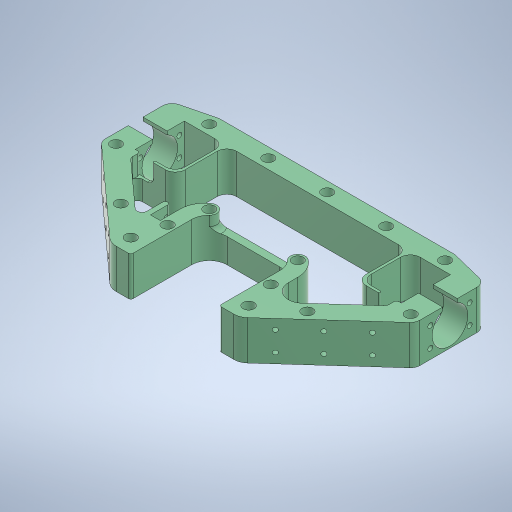
# Autodesk Inventor part: Chassis
Saved by Autodesk Inventor 2023.2 (Build 272271000, 271)
## iProperties
Created: 2022-05-26
Part Number: Chassis
Material: Nylon 6/6
Document SubType Name: Modeling
Designer: Nathan Cai
Density: 0.861189 g/cm^3
Appearance: Smooth - Dark Sea Green
Mass: 131.31 g
Surface Area: 564.609 cm^2
Volume: 152.475 cm^3
Author: Nathan Cai
Autodesk Inventor part; units mm, degrees
ref_plane "YZ Plane" through (0, 0, 0) normal (1, 0, 0) x (0, 1, 0)
ref_plane "XZ Plane" through (0, 0, 0) normal (0, 1, 0) x (-1, 0, 0)
ref_plane "XY Plane" through (0, 0, 0) normal (0, 0, 1) x (1, 0, 0)
sketch "Sketch1" plane through (0, 0, 0) normal (0, 1, 0) x (-1, 0, 0)
  line L0 (101.6, 38.1) -> (-101.6, 38.1) construction
  line L1 (-101.6, 38.1) -> (-101.6, -38.1) construction
  line L2 (-101.6, -38.1) -> (101.6, -38.1)
  line L3 (101.6, -38.1) -> (101.6, 38.1) construction
  line L4 (101.6, 38.1) -> (-101.6, -38.1) construction
  line L5 (-101.6, 38.1) -> (101.6, -38.1) construction
  line L6 (-28.575, 66.675) -> (28.575, 66.675) construction
  line L7 (28.575, 66.675) -> (28.575, 9.525)
  line L8 (28.575, 9.525) -> (-28.575, 9.525)
  line L9 (-28.575, 9.525) -> (-28.575, 66.675)
  line L10 (-28.575, 66.675) -> (28.575, 9.525) construction
  line L11 (28.575, 66.675) -> (-28.575, 9.525) construction
  circle A0 centre (-38.1, 50.8) radius 3.556
  line L12 (0, 38.1) -> (0, -38.1) construction
  circle A1 centre (-38.1, 50.8) radius 9.525
  line L13 (-38.1, 60.325) -> (-28.575, 60.325)
  circle A2 centre (38.1, 50.8) radius 3.556
  circle A3 centre (38.1, 50.8) radius 9.525
  line L14 (38.1, 60.325) -> (28.575, 60.325)
  circle A4 centre (-76.2, -38.1) radius 3.4925
  circle A5 centre (-95.25, 3.175) radius 3.4925
  circle A6 centre (76.2, -38.1) radius 3.4925
  circle A7 centre (95.25, 3.175) radius 3.4925
  line L15 (-101.6, -38.1) -> (-101.6, 6.35)
  line L16 (-101.6, 6.35) -> (-44.479723, 57.872818)
  line L17 (101.6, -38.1) -> (101.6, 6.35)
  line L18 (101.6, 6.35) -> (44.479723, 57.872818)
  line L19 (-42.641743, 42.427533) -> (-86.025, 3.295586)
  line L20 (-86.025, 3.295586) -> (-86.025, -38.1)
  line L21 (86.025, -38.1) -> (86.025, 3.295586)
  line L22 (86.025, 3.295586) -> (42.641743, 42.427533)
  line L23 (0, -38.1) -> (-95.25, -38.1)
  line L24 (0, -38.1) -> (95.25, -38.1) construction
  circle A8 centre (-60.325, 35.028711) radius 3.4925
  circle A9 centre (-33.3375, 31.75) radius 3.4925
  line L25 (-38.1, 0) -> (-38.1, 41.275)
  line L26 (-38.1, 0) -> (0, 0) construction
  circle A10 centre (60.325, 35.028711) radius 3.4925
  circle A11 centre (33.3375, 31.75) radius 3.4925
  line L27 (38.1, 0) -> (38.1, 41.275)
  line L28 (38.1, 0) -> (0, 0) construction
  line L29 (-86.025, 0) -> (-60.1, 0)
  line L30 (-60.1, 0) -> (-60.1, -31.75)
  line L31 (-60.1, -31.75) -> (-87.975, -31.75)
  line L32 (-101.6, -38.1) -> (101.6, -38.1) construction
  line L33 (101.6, -38.1) -> (101.6, 19.05)
  line L34 (101.6, 19.05) -> (-101.6, 19.05) construction
  line L35 (-101.6, 19.05) -> (-101.6, -38.1)
  line L36 (-101.6, 19.05) -> (-87.520267, 19.05) construction
  line L37 (87.520267, 19.05) -> (101.6, 19.05) construction
  circle A12 centre (-38.1, 0) radius 3.175 construction
  circle A13 centre (-38.1, 0) radius 6.35 construction
  circle A14 centre (38.1, 0) radius 3.175 construction
  circle A15 centre (38.1, 0) radius 6.35 construction
  circle A16 centre (28.575, 9.525) radius 3.4925
  circle A17 centre (28.575, 9.525) radius 4.7625
  arc A18 (17.077308, 9.525) -> (28.575, 21.022692) centre (17.077308, 21.022692) ccw
  circle A19 centre (-28.575, 9.525) radius 3.4925
  circle A20 centre (-28.575, 9.525) radius 4.7625
  arc A21 (-28.575, 21.022692) -> (-17.077308, 9.525) centre (-17.077308, 21.022692) ccw
  arc A22 (31.4325, 5.715) -> (38.1, 19.05) centre (21.43125, 19.05) ccw
  arc A23 (-38.1, 19.05) -> (-31.4325, 5.715) centre (-21.43125, 19.05) ccw
  line L38 (-58.5125, -38.1) -> (-58.5125, 28.112019)
  line L39 (86.025, 0) -> (60.1, 0)
  line L40 (60.1, 0) -> (60.1, -31.75)
  line L41 (60.1, -31.75) -> (87.975, -31.75)
  line L42 (58.5125, -38.1) -> (58.5125, 28.112019)
  line L43 (-28.575, 4.7625) -> (28.575, 4.7625)
  line L44 (101.6, -31.75) -> (-101.6, -31.75)
  line L45 (-101.6, -31.75) -> (-101.6, -44.45) construction
  line L46 (-101.6, -44.45) -> (101.6, -44.45)
  line L47 (101.6, -44.45) -> (101.6, -31.75) construction
  circle A24 centre (0, -38.1) radius 3.4925
  circle A25 centre (38.1, -38.1) radius 3.4925
  circle A26 centre (-38.1, -38.1) radius 3.4925
  line L48 (101.6, -38.1) -> (76.2, -44.45)
  line L49 (-101.6, -38.1) -> (-76.2, -44.45)
  line L50 (76.2, -38.1) -> (76.2, -44.45) construction
  line L51 (-76.2, -38.1) -> (-76.2, -44.45) construction
  line L52 (-58.5125, 1.5875) -> (-87.918653, 1.5875)
  line L53 (58.5125, 1.5875) -> (87.918653, 1.5875)
  line L54 (38.1, 19.05) -> (44.45, 19.05)
  line L55 (44.45, 19.05) -> (44.45, 31.75)
  line L56 (44.45, 31.75) -> (38.1, 31.75)
  line L57 (38.1, 31.75) -> (38.1, 19.05)
  line L58 (38.1, 19.05) -> (47.625, 19.05)
  line L59 (47.625, 19.05) -> (47.625, 37.932607)
  line L60 (47.625, 37.932607) -> (38.1, 37.932607) construction
  line L61 (38.1, 37.932607) -> (38.1, 19.05)
  point P0 (28.575, 38.1)
  point P1 (-28.575, 38.1)
  point P2 (28.575, 60.325)
  point P3 (44.479723, 57.872818)
  point P4 (101.6, -15.875)
  point P5 (38.1, 41.275)
  point P6 (-86.025, -31.75)
  point P7 (-101.6, 6.35)
  point P8 (101.6, 6.35)
  point P9 (31.75, 0)
  point P10 (38.1, 6.35)
  point P11 (-38.1, 6.35)
  point P12 (-31.75, 0)
  point P13 (86.025, -31.75)
  point P14 (86.025, 0)
  point P15 (58.5125, 28.112019)
  point P16 (-17.077308, 9.525)
  point P17 (-28.575, 21.022692)
  point P18 (-38.1, 19.05)
  point P19 (-31.4325, 5.715)
  point P20 (-21.850242, 0)
  point P21 (21.850242, 0)
  point P22 (-25.207404, 12.892596)
  point P23 (-28.575, 14.2875)
  point P24 (-23.8125, 9.525)
  point P25 (-28.575, 50.8)
  point P26 (25.207404, 12.892596)
  point P27 (28.575, 14.2875)
  point P28 (23.8125, 9.525)
  point P29 (28.575, 50.8)
  point P30 (25.0825, 9.525)
  point P31 (28.575, 13.0175)
  point P32 (58.5125, -31.75)
  point P33 (-58.5125, -31.75)
  point P34 (87.918653, 1.5875)
  point P35 (58.5125, 1.5875)
  point P36 (86.025, -31.75)
  point P37 (86.025, 1.5875)
  point P38 (-86.025, 1.5875)
  point P39 (-86.025, -31.75)
  point P40 (-34.6075, -38.1)
  point P41 (-41.5925, -38.1)
  point P42 (-3.4925, -38.1)
  point P43 (3.4925, -38.1)
  point P44 (41.5925, -38.1)
  point P45 (34.6075, -38.1)
  point P46 (-72.7075, -38.1)
  point P47 (-79.6925, -38.1)
  dimension "d166" = 12.7
  dimension "d169" = 22.225
  dimension "d0" = 203.2
  dimension "d1" = 76.2
  dimension "d4" = 57.15
  dimension "d6" = 7.112
  dimension "d7" = 38.1
  dimension "d8" = 19.05
  dimension "d10" = 6.985
  dimension "d11" = 6.985
  dimension "d12" = 0
  dimension "d14" = 25.4
  dimension "d15" = 6.35
  dimension "d20" = 50.8
  dimension "d21" = 41.275
  dimension "d22" = 44.45
  dimension "d24" = 12.7
  dimension "d25" = 15.575
  dimension "d26" = 12.7
  dimension "d27" = 15.575
  dimension "d31" = 6.985
  dimension "d32" = 6.985
  dimension "d33" = 6.35
  dimension "d34" = 31.75
  dimension "d35" = 4.7625
  dimension "d36" = 22.225
  dimension "d37" = 9.525
  dimension "d39" = 31.75
  dimension "d40" = 6.35
  dimension "d42" = 57.15
  dimension "d43" = 6.35
  dimension "d44" = 9.525
  dimension "d45" = 9.525
  dimension "d46" = 12.7
  dimension "d104" = 6.985
  dimension "d105" = 9.525
  dimension "d106" = 1.5875
  dimension "d123" = 88.9
  dimension "d124" = 12.7
  dimension "d125" = 6.985
  dimension "d126" = 6.985
  dimension "d127" = 38.1
  dimension "d128" = 28.575
  dimension "d134" = 1.5875
  dimension "d137" = 6.35
  dimension "d138" = 12.7
  dimension "d139" = 9.525
  dimension "d178" = 41.5
  constraints: 125 end point, 32 symmetric about line, 26 centre point, 25 point on line, 16 parallel, 16 point on circle, 11 horizontal, 9 perpendicular, 8 midpoint, 8 tangent, 7 coincident, 2 vertical, 1 collinear, 16 other
  measures "d0" distance of L2.end L1.end
  measures "d1" distance between parallel lines of L0 L2
  measures "d4" distance of L7.end L8.end
  measures "d6" diameter of A0
  measures "d7" distance from line of L12 A0.centre
  measures "d8" diameter of A1
  measures "d10" diameter of A4
  measures "d11" diameter of A5
  measures "d12" distance from line of L2 L51.start
  measures "d14" distance from line of L1 L51.start
  measures "d15" distance from line of L1 A5.centre
  measures "d20" distance between parallel lines of L8 L14
  measures "d21" vertical distance of L51.start A5.centre
  measures "d22" distance of L1.end L15.end
  measures "d24" distance between parallel lines of L16 L19
  measures "d25" distance between parallel lines of L15 L20
  measures "d26" distance between parallel lines of L18 L22
  measures "d27" distance from line of point (101.6, -15.875) L21
  measures "d31" diameter of A8
  measures "d32" diameter of A9
  measures "d33" distance from line of L16 A8.centre
  measures "d34" distance from line of L9 A8.centre
  measures "d35" distance from line of L9 A9.centre
  measures "d36" distance from line of L8 A9.centre
  measures "d37" distance between parallel lines of L9 L25
  measures "d39" distance between parallel lines of L31 L29
  measures "d40" distance between parallel lines of L23 L31
  measures "d42" distance of L33.end L32.end
  measures "d43" diameter of A12
  measures "d44" distance from line of L8 A12.centre
  measures "d45" distance from line of L9 A12.centre
  measures "d46" diameter of A13
  measures "d104" diameter of A16
  measures "d105" diameter of A17
  measures "d106" distance between parallel lines of L30 L38
  measures "d123" distance from line of L32 A1.centre
  measures "d124" distance between parallel lines of L44 L46
  measures "d125" diameter of A24
  measures "d126" diameter of A25
  measures "d127" distance of A24.centre A25.centre
  measures "d128" distance from line of L12 A16.centre
  measures "d134" distance between parallel lines of L29 L52
  measures "d137" distance of L56.end L55.end
  measures "d138" distance of L55.end L54.end
  measures "d139" distance of L60.end L59.end
  measures "d178" distance between parallel lines of L1 L30
extrude "Extrusion1" add sketch "Sketch1" along normal blind 25.4 contours L15 L44 L31 L20 L2 | L2 A4 A26 A24 A25 A6 L48 L46 L49 | L15 L16 A1 L19 L20 L31 L44 | L20 L31 L44 L38 L2 A4 | A1 | L2 L21 L41 L44 L17 | L20 L52 L38 L44 L30 L29 | L13 L9 A1 | L2 A6 L42 L44 L41 L21 | L44 L41 L21 L22 A3 L18 L17 | L38 L44 L42 L2 A25 A24 A26 | L9 A20 A23 L25 A1 | L42 L53 L21 L39 L40 L44 | A21 A20 L9 | A3 | A20 L8 A19 L9 | L9 A19 L8 A20 | A21 L8 A20 | A3 L7 L14 | L8 A17 L43 A20 | L22 L59 L58 L55 L56 L27 A3 | A3 L27 A22 A17 L7 | A18 A17 L8 | A17 L8 A16 L7 | L7 A17 A18 | A17 L7 A16 L8 | L54 L27 L56 L55
fillet "Fillet1" radius 6.35 14 edges at (60.1, 12.7, 0) (60.1, 12.7, -31.75) (101.6, 12.7, -38.1) (101.6, 12.7, 6.35) (-101.6, 12.7, 6.35) (-60.1, 12.7, -31.75) (-60.1, 12.7, 0) (-58.5125, 12.7, -31.75) (58.5125, 12.7, -31.75) (76.2, 12.7, -44.45) (-76.2, 12.7, -44.45) (-101.6, 12.7, -38.1) (58.5125, 12.7, 1.5875) (-58.5125, 12.7, 1.5875)
sketch "Sketch2" plane through (0, 25.4, 0) normal (0, 1, 0) x (1, 0, 0)
  line L0 (-38.1, -19.05) -> (-47.625, -19.05) projected
  line L1 (-38.1, -19.05) -> (-44.45, -19.05)
  line L2 (-44.45, -19.05) -> (-44.45, -31.75)
  line L3 (-44.45, -31.75) -> (-38.1, -31.75)
  line L4 (-38.1, -31.75) -> (-38.1, -19.05)
  point P0 (0, 0)
  dimension "d140" = 6.35
  dimension "d141" = 12.7
  constraints: 8 end point, 2 parallel, 1 horizontal, 1 perpendicular
  measures "d140" distance of L3.end L2.end
  measures "d141" distance of L2.end L1.end
extrude "Extrusion2" cut sketch "Sketch2" against normal blind 12.7
fillet "Fillet2" [suppressed]
sketch "Sketch3" plane through (101.6, 0, 15.875) normal (1, 0, 0) x (0, 0, -1)
  circle A0 centre (31.75, 12.7) radius 11.5
  line L0 (0, 25.4) -> (50.8, 25.4) projected
  line L1 (50.8, 0) -> (50.8, 25.4) projected
  circle A1 centre (19.05, 6.35) radius 1.5875
  line L2 (0, 0) -> (50.8, 0) projected
  circle A2 centre (44.45, 6.35) radius 1.5875
  circle A3 centre (19.05, 19.05) radius 1.5875
  circle A4 centre (44.45, 19.05) radius 1.5875
  point P0 (15.875, 0)
  dimension "d54" = 23
  dimension "d55" = 12.7
  dimension "d56" = 19.05
  dimension "d63" = 3.175
  dimension "d64" = 6.35
  dimension "d65" = 12.7
  dimension "d68" = 25.4
  dimension "d71" = 12.7
  constraints: 5 centre point, 1 horizontal, 1 vertical, 6 other
  measures "d54" diameter of A0
  measures "d55" distance from line of L0 A0.centre
  measures "d56" distance from line of L1 A0.centre
  measures "d63" diameter of A1
  measures "d64" distance from line of L2 A1.centre
  measures "d65" horizontal distance of A0.centre A1.centre
  measures "d68" distance of A1.centre A2.centre
  measures "d71" distance of A1.centre A3.centre
extrude "Extrusion3" cut sketch "Sketch3" against normal blind 19.05
sketch "Sketch4" plane through (0, 25.4, 0) normal (0, 1, 0) x (1, 0, 0)
  line L0 (101.6, 11.1125) -> (86.025, 11.1125)
  line L1 (86.025, 11.1125) -> (86.025, 20.6375)
  line L2 (86.025, 20.6375) -> (101.6, 20.6375)
  line L3 (101.6, 20.6375) -> (101.6, 11.1125)
  line L4 (44.45, 47.625) -> (-44.45, 47.625)
  line L5 (66.45, 31.75) -> (86.025, 31.75)
  line L6 (86.025, 0) -> (66.45, 0)
  line L7 (58.5125, 25.4) -> (58.5125, 4.7625)
  line L8 (86.025, 0) -> (58.5125, 0)
  line L9 (58.5125, 0) -> (58.5125, -12.7)
  line L10 (58.5125, -12.7) -> (86.025, -12.7)
  line L11 (86.025, -12.7) -> (86.025, 0) construction
  line L12 (86.025, -12.7) -> (82.85, -12.7)
  line L13 (82.85, -12.7) -> (82.85, 0)
  line L14 (82.85, 0) -> (86.025, 0)
  line L15 (86.025, 0) -> (86.025, -12.7) construction
  line L16 (86.025, -3.295586) -> (42.641743, -42.427533)
  line L17 (75.598887, -12.7) -> (82.85, -6.159454)
  line L18 (73.325, 0) -> (73.325, -12.7)
  point P0 (0, 0)
  point P1 (88.9, 47.625)
  point P2 (-88.9, 47.625)
  point P3 (101.6, 33.14207)
  point P4 (61.94, 31.75)
  point P5 (61.94, -22.196554)
  point P6 (82.85, 0)
  point P7 (61.94, 0)
  point P8 (58.5125, 0)
  point P9 (81.784983, -7.120106)
  point P10 (73.325, 0)
  point P11 (58.5125, -28.112019)
  point P12 (82.85, -6.159454)
  dimension "d59" = 9.525
  dimension "d60" = 26.9875
  dimension "d112" = 12.7
  dimension "d113" = 3.175
  dimension "d135" = 9.525
  constraints: 28 end point, 8 point on line, 6 parallel, 4 perpendicular, 3 horizontal, 1 collinear, 2 other
  measures "d59" distance of L0.end L1.end
  measures "d60" distance between parallel lines of L4 L2
  measures "d112" distance of L9.end L8.end
  measures "d113" distance of L13.end L14.end
  measures "d135" distance between parallel lines of L13 L18
extrude "Extrusion4" cut sketch "Sketch4" against normal blind 12.7 contours L0 L1 L2 L3 | L13 L16 L10 L18 L6
ref_plane "Work Plane1" through (0, 0, 53.975) normal (1, 0, 0) x (0, 0, -1)
fillet "Fillet9" radius 3.175 4 edges at (86.025, 12.7, 1.5875) (86.025, 12.7, 3.2956) (-86.025, 12.7, 3.2956) (-86.025, 12.7, 1.5875)
mirror "Mirror1" about plane through (0, 0, 53.975) normal (1, 0, 0) of "Extrusion3", "Extrusion4"
fillet "Fillet3" radius 1.5875 4 edges at (82.85, 19.05, 0) (-82.85, 19.05, 0) (-44.45, 19.05, 19.05) (-47.625, 12.7, 19.05)
fillet "Fillet4" radius 9.525 2 edges at (38.1, 12.7, 41.275) (42.6417, 12.7, 42.4275)
fillet "Fillet5" radius 1.5875 2 edges at (-28.575, 12.7, 60.325) (28.575, 12.7, 60.325)
fillet "Fillet6" radius 3.175 1 edges at (-47.625, 12.7, 37.9326)
fillet "Fillet10" radius 3.175 2 edges at (82.85, 19.05, 6.1595) (-82.85, 19.05, 6.1595)
sketch "Sketch8" plane through (-47.625, 0, 20.6375) normal (-1, 0, 0) x (0, 0, 1)
  point P0 (0.9525, 19.05)
  point P1 (8.5725, 19.05)
hole "Hole2" at (-47.625, 19.05, 21.59) at (-47.625, 19.05, 29.21) direction (1, 0, 0) diameter 2.4384 depth 3.175
sketch "Sketch10" plane through (-44.479723, 0, 57.872818) normal (-0.6697872, 0, 0.7425531) x (0.7425531, 0, 0.6697872)
  line L0 (-74.100323, 0) -> (-74.100323, 25.4) construction
  line L1 (-74.100323, 0) -> (0, 0) construction
  line L2 (-74.100323, 25.4) -> (0, 25.4) construction
  line L3 (0, 25.4) -> (0, 0) construction
  line L4 (0, 0) -> (-74.100323, 0) construction
  line L5 (-74.100323, 0) -> (-74.100323, 25.4) construction
  line L6 (-74.100323, 25.4) -> (0, 25.4)
  line L7 (-57.15, 25.4) -> (-57.15, 0) construction
  line L8 (-12.7, 25.4) -> (-12.7, 0) construction
  line L9 (0, 0) -> (0, 25.4)
  line L10 (-78.815535, 25.4) -> (-78.815535, 0)
  line L11 (-34.925, 25.4) -> (-34.925, 0) construction
  line L12 (-57.15, 12.7) -> (-12.7, 12.7) construction
  line L13 (-57.15, 19.05) -> (-12.7, 19.05) construction
  line L14 (-57.15, 6.35) -> (-12.7, 6.35) construction
  circle A0 centre (-57.15, 19.05) radius 1.389063
  circle A1 centre (-57.15, 6.35) radius 1.389063
  circle A2 centre (-34.925, 19.05) radius 1.389063
  circle A3 centre (-34.925, 6.35) radius 1.389063
  circle A4 centre (-12.7, 19.05) radius 1.389063
  circle A5 centre (-12.7, 6.35) radius 1.389063
  point P0 (-5.733915, 0)
  dimension "d157" = 12.7
  dimension "d158" = 44.45
  dimension "d159" = 22.225
  dimension "d161" = 6.35
  dimension "d162" = 6.35
  dimension "d163" = 2.77813
  dimension "d166" = 12.7
  dimension "d169" = 22.225
  constraints: 20 end point, 7 point on line, 6 centre point, 6 parallel, 3 perpendicular, 2 horizontal, 2 midpoint, 1 coincident, 1 vertical, 10 other
  measures "d157" distance between parallel lines of L3 L8
  measures "d158" distance between parallel lines of L7 L8
  measures "d159" distance between parallel lines of L8 L11
  measures "d161" distance between parallel lines of L12 L13
  measures "d162" distance between parallel lines of L12 L14
  measures "d163" diameter of A0
  measures "d166" distance of A0.centre A1.centre
  measures "d169" distance of A0.centre A2.centre
extrude "Extrusion7" cut sketch "Sketch10" against normal blind 12.7
mirror "Mirror3" about plane through (0, 0, 53.975) normal (1, 0, 0) of "Extrusion7"
fillet "Fillet7" radius 0.79375 4 edges at (73.325, 19.05, 1.5875) (73.325, 19.05, 0) (-73.325, 19.05, 1.5875) (-73.325, 19.05, 0)
sketch "Sketch11" plane through (0, 25.4, 0) normal (0, 1, 0) x (1, 0, 0)
  circle A0 centre (28.575, -9.525) radius 3.4925
  arc A1 (31.4325, -5.715) -> (28.575, -4.7625) centre (28.575, -9.525) ccw
  circle A2 centre (28.575, -9.525) radius 4.7625
  arc A3 (-28.575, -4.7625) -> (-31.4325, -5.715) centre (-28.575, -9.525) ccw
  circle A4 centre (-28.575, -9.525) radius 4.7625
  arc A5 (28.575, -58.7375) -> (30.1625, -60.325) centre (30.1625, -58.7375) ccw
  line L0 (30.1625, -60.325) -> (38.1, -60.325)
  arc A6 (38.1, -60.325) -> (44.479723, -57.872818) centre (38.1, -50.8) ccw
  line L1 (44.479723, -57.872818) -> (99.503149, -8.241372)
  arc A7 (99.503149, -8.241372) -> (101.6, -3.52616) centre (95.25, -3.52616) ccw
  line L2 (101.6, -3.52616) -> (101.6, 11.1125)
  line L3 (101.6, 11.1125) -> (86.025, 11.1125)
  line L4 (86.025, 11.1125) -> (86.025, 0)
  line L5 (86.025, 0) -> (84.4375, 0)
  arc A8 (84.4375, 0) -> (82.85, -1.5875) centre (84.4375, -1.5875) ccw
  line L6 (82.85, -4.747534) -> (82.85, -1.5875)
  line L7 (81.801574, -7.10514) -> (54.004723, -32.17806)
  arc A9 (38.1, -25.105242) -> (54.004723, -32.17806) centre (47.625, -25.105242) ccw
  line L8 (38.1, -25.105242) -> (38.1, -19.05)
  arc A10 (38.1, -19.05) -> (31.4325, -5.715) centre (21.43125, -19.05) ccw
  arc A11 (31.4325, -5.715) -> (28.575, -4.7625) centre (28.575, -9.525) ccw
  line L9 (28.575, -4.7625) -> (-28.575, -4.7625)
  arc A12 (-28.575, -4.7625) -> (-31.4325, -5.715) centre (-28.575, -9.525) ccw
  arc A13 (-31.4325, -5.715) -> (-38.1, -19.05) centre (-21.43125, -19.05) ccw
  line L10 (-38.1, -19.05) -> (-38.1, -31.75)
  line L11 (-38.1, -31.75) -> (-44.45, -31.75)
  line L12 (-47.625, -20.6375) -> (-47.625, -30.79295)
  arc A14 (-52.926574, -33.150556) -> (-47.625, -30.79295) centre (-50.8, -30.79295) ccw
  line L13 (-52.926574, -33.150556) -> (-81.801574, -7.10514)
  line L14 (-82.85, -4.747534) -> (-82.85, -1.5875)
  arc A15 (-82.85, -1.5875) -> (-84.4375, 0) centre (-84.4375, -1.5875) ccw
  line L15 (-84.4375, 0) -> (-86.025, 0)
  line L16 (-86.025, 0) -> (-86.025, 11.1125)
  line L17 (-86.025, 11.1125) -> (-101.6, 11.1125)
  line L18 (-101.6, 11.1125) -> (-101.6, -3.52616)
  arc A16 (-101.6, -3.52616) -> (-99.503149, -8.241372) centre (-95.25, -3.52616) ccw
  line L19 (-99.503149, -8.241372) -> (-44.479723, -57.872818)
  arc A17 (-44.479723, -57.872818) -> (-38.1, -60.325) centre (-38.1, -50.8) ccw
  line L20 (-38.1, -60.325) -> (-30.1625, -60.325)
  arc A18 (-30.1625, -60.325) -> (-28.575, -58.7375) centre (-30.1625, -58.7375) ccw
  line L21 (-28.575, -58.7375) -> (-28.575, -21.022692)
  arc A19 (-17.077308, -9.525) -> (-28.575, -21.022692) centre (-17.077308, -21.022692) ccw
  line L22 (-17.077308, -9.525) -> (17.077308, -9.525)
  arc A20 (28.575, -21.022692) -> (17.077308, -9.525) centre (17.077308, -21.022692) ccw
  line L23 (28.575, -21.022692) -> (28.575, -58.7375)
  circle A21 centre (38.1, -50.8) radius 3.556
  circle A22 centre (60.325, -35.028711) radius 3.4925
  circle A23 centre (95.25, -3.175) radius 3.4925
  circle A24 centre (-33.3375, -31.75) radius 3.4925
  circle A25 centre (-28.575, -9.525) radius 3.4925
  circle A26 centre (33.3375, -31.75) radius 3.4925
  circle A27 centre (28.575, -9.525) radius 3.4925
  circle A28 centre (-60.325, -35.028711) radius 3.4925
  circle A29 centre (-95.25, -3.175) radius 3.4925
  circle A30 centre (-38.1, -50.8) radius 3.556
  line L24 (86.025, 20.6375) -> (101.6, 20.6375)
  line L25 (101.6, 20.6375) -> (101.6, 33.14207)
  arc A31 (101.6, 33.14207) -> (96.790101, 39.302475) centre (95.25, 33.14207) ccw
  line L26 (96.790101, 39.302475) -> (76.95838, 44.260405)
  arc A32 (76.95838, 44.260405) -> (75.418279, 44.45) centre (75.418279, 38.1) ccw
  line L27 (75.418279, 44.45) -> (-75.418279, 44.45)
  arc A33 (-75.418279, 44.45) -> (-76.95838, 44.260405) centre (-75.418279, 38.1) ccw
  line L28 (-76.95838, 44.260405) -> (-96.790101, 39.302475)
  arc A34 (-96.790101, 39.302475) -> (-101.6, 33.14207) centre (-95.25, 33.14207) ccw
  line L29 (-101.6, 33.14207) -> (-101.6, 20.6375)
  line L30 (-101.6, 20.6375) -> (-86.025, 20.6375)
  line L31 (-58.5125, 4.7625) -> (-58.5125, 25.4)
  line L32 (-52.1625, 31.75) -> (52.1625, 31.75)
  arc A35 (-60.1, 25.4) -> (-66.45, 31.75) centre (-66.45, 25.4) ccw
  line L33 (-60.1, 25.4) -> (-60.1, 6.35)
  arc A36 (-66.45, 0) -> (-60.1, 6.35) centre (-66.45, 6.35) ccw
  line L34 (58.5125, 25.4) -> (58.5125, 4.7625)
  arc A37 (81.801574, -7.10514) -> (82.85, -4.747534) centre (79.675, -4.747534) ccw
  arc A38 (-44.45, -20.6375) -> (-47.625, -20.6375) centre (-46.0375, -20.6375) ccw
  arc A39 (-82.85, -4.747534) -> (-81.801574, -7.10514) centre (-79.675, -4.747534) ccw
  arc A40 (-72.53125, 0) -> (-72.53125, -1.5875) centre (-72.53125, -0.79375) ccw
  line L35 (-72.53125, -1.5875) -> (-64.8625, -1.5875)
  arc A41 (-64.8625, -1.5875) -> (-58.5125, 4.7625) centre (-64.8625, 4.7625) ccw
  arc A42 (-52.1625, 31.75) -> (-58.5125, 25.4) centre (-52.1625, 25.4) ccw
  arc A43 (58.5125, 25.4) -> (52.1625, 31.75) centre (52.1625, 25.4) ccw
  arc A44 (58.5125, 4.7625) -> (64.8625, -1.5875) centre (64.8625, 4.7625) ccw
  line L36 (64.8625, -1.5875) -> (72.53125, -1.5875)
  arc A45 (72.53125, -1.5875) -> (72.53125, 0) centre (72.53125, -0.79375) ccw
  line L37 (72.53125, 0) -> (66.45, 0)
  arc A46 (60.1, 6.35) -> (66.45, 0) centre (66.45, 6.35) ccw
  line L38 (60.1, 6.35) -> (60.1, 25.4)
  arc A47 (66.45, 31.75) -> (60.1, 25.4) centre (66.45, 25.4) ccw
  line L39 (66.45, 31.75) -> (86.025, 31.75)
  line L40 (86.025, 31.75) -> (86.025, 20.6375)
  line L41 (-86.025, 20.6375) -> (-86.025, 31.75)
  line L42 (-86.025, 31.75) -> (-66.45, 31.75)
  line L43 (-66.45, 0) -> (-72.53125, 0)
  circle A48 centre (76.2, 38.1) radius 3.4925
  circle A49 centre (-38.1, 38.1) radius 3.4925
  circle A50 centre (0, 38.1) radius 3.4925
  circle A51 centre (38.1, 38.1) radius 3.4925
  line L44 (-44.45, -31.75) -> (-44.45, -20.6375)
  point P0 (0, 0)
  point P1 (25.207404, -12.892596)
  point P2 (28.575, -4.7625)
  point P3 (-28.575, -4.7625)
  point P4 (-25.207404, -12.892596)
  constraints: 2 coincident, 6 other
extrude "Extrusion8" cut sketch "Sketch11" against normal blind 9.525 contours A2 A20 L22 A19 A4 L9
fillet "Fillet8" radius 3.175 4 edges at (-24.175, 15.875, 7.7025) (24.175, 15.875, 7.7025) (73.325, 12.7, 0.7937) (-73.325, 12.7, 0.7938)
equation "\"d35\" = 0.5 * d37"
body "Solid1"
